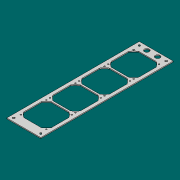
# Autodesk Inventor part: front_panel
Saved by Autodesk Inventor 2018.2 (Build 222227000, 227)
## iProperties
Created: 2019-10-14
Part Number: front_panel
Material: アルミニウム 6061
Document SubType Name: Modeling
Designer: gisen
Density: 2.7 g/cm^3
Appearance: アルミニウム - フラット
Author: gisen
Autodesk Inventor part; units mm, degrees
ref_plane "YZ Plane" through (0, 0, 0) normal (1, 0, 0) x (0, 1, 0)
ref_plane "XZ Plane" through (0, 0, 0) normal (0, 1, 0) x (-1, 0, 0)
ref_plane "XY Plane" through (0, 0, 0) normal (0, 0, 1) x (1, 0, 0)
sketch "スケッチ1" plane through (0, 0, 0) normal (0, 0, 1) x (1, 0, 0)
  line L0 (-55, -215) -> (55, -215)
  line L1 (55, -215) -> (55, 215)
  line L2 (55, 215) -> (-55, 215)
  line L3 (-55, 215) -> (-55, -215)
  line L4 (-55, -215) -> (55, 215) construction
  line L5 (55, -215) -> (-55, 215) construction
  line L6 (-55, 185) -> (-50, 185) construction
  line L7 (-50, 185) -> (-25, 210) construction
  line L8 (-25, 210) -> (-25, 215) construction
  line L9 (-46, 95.75) -> (46, 95.75) construction
  line L10 (46, 95.75) -> (46, 187.75) construction
  line L11 (46, 187.75) -> (-46, 187.75) construction
  line L12 (-46, 187.75) -> (-46, 95.75) construction
  line L13 (-46, 95.75) -> (46, 187.75) construction
  line L14 (46, 95.75) -> (-46, 187.75) construction
  line L15 (-46, 1.25) -> (46, 1.25) construction
  line L16 (46, 1.25) -> (46, 93.25) construction
  line L17 (46, 93.25) -> (-46, 93.25) construction
  line L18 (-46, 93.25) -> (-46, 1.25) construction
  line L19 (-46, 1.25) -> (46, 93.25) construction
  line L20 (46, 1.25) -> (-46, 93.25) construction
  line L21 (0, 0) -> (0, 141.75) construction
  circle A0 centre (0, 141.75) radius 53 construction
  line L22 (-44.7, 97.05) -> (44.7, 97.05) construction
  line L23 (44.7, 97.05) -> (44.7, 186.45) construction
  line L24 (44.7, 186.45) -> (-44.7, 186.45) construction
  line L25 (-44.7, 186.45) -> (-44.7, 97.05) construction
  line L26 (-44.7, 97.05) -> (44.7, 186.45) construction
  line L27 (44.7, 97.05) -> (-44.7, 186.45) construction
  arc A1 (-28.4765, 186.45) -> (-44.7, 170.2265) centre (0, 141.75) ccw
  arc A2 (-44.7, 113.2735) -> (-28.4765, 97.05) centre (0, 141.75) ccw
  arc A3 (28.4765, 97.05) -> (44.7, 113.2735) centre (0, 141.75) ccw
  arc A4 (44.7, 170.2265) -> (28.4765, 186.45) centre (0, 141.75) ccw
  line L28 (-28.4765, 186.45) -> (28.4765, 186.45)
  line L29 (-44.7, 170.2265) -> (-44.7, 113.2735)
  line L30 (-28.4765, 97.05) -> (28.4765, 97.05)
  line L31 (44.7, 113.2735) -> (44.7, 170.2265)
  line L32 (-41.25, 100.5) -> (41.25, 100.5) construction
  line L33 (41.25, 100.5) -> (41.25, 183) construction
  line L34 (41.25, 183) -> (-41.25, 183) construction
  line L35 (-41.25, 183) -> (-41.25, 100.5) construction
  line L36 (-41.25, 100.5) -> (41.25, 183) construction
  line L37 (41.25, 100.5) -> (-41.25, 183) construction
  circle A5 centre (-41.25, 183) radius 2.25
  circle A6 centre (-41.25, 100.5) radius 2.25
  circle A7 centre (41.25, 100.5) radius 2.25
  circle A8 centre (41.25, 183) radius 2.25
  circle A9 centre (-41.25, 88.5) radius 2.25
  arc A10 (-28.4765, 91.95) -> (-44.7, 75.7265) centre (0, 47.25) ccw
  line L38 (-28.4765, 91.95) -> (28.4765, 91.95)
  arc A11 (44.7, 75.7265) -> (28.4765, 91.95) centre (0, 47.25) ccw
  circle A12 centre (41.25, 88.5) radius 2.25
  line L39 (44.7, 18.7735) -> (44.7, 75.7265)
  arc A13 (28.4765, 2.55) -> (44.7, 18.7735) centre (0, 47.25) ccw
  circle A14 centre (41.25, 6) radius 2.25
  line L40 (-28.4765, 2.55) -> (28.4765, 2.55)
  circle A15 centre (-41.25, 6) radius 2.25
  arc A16 (-44.7, 18.7735) -> (-28.4765, 2.55) centre (0, 47.25) ccw
  line L41 (-44.7, 75.7265) -> (-44.7, 18.7735)
  circle A17 centre (-41.25, -6) radius 2.25
  arc A18 (-28.4765, -2.55) -> (-44.7, -18.7735) centre (0, -47.25) ccw
  line L42 (-28.4765, -2.55) -> (28.4765, -2.55)
  arc A19 (44.7, -18.7735) -> (28.4765, -2.55) centre (0, -47.25) ccw
  circle A20 centre (41.25, -6) radius 2.25
  line L43 (44.7, -75.7265) -> (44.7, -18.7735)
  arc A21 (28.4765, -91.95) -> (44.7, -75.7265) centre (0, -47.25) ccw
  circle A22 centre (41.25, -88.5) radius 2.25
  line L44 (-28.4765, -91.95) -> (28.4765, -91.95)
  circle A23 centre (-41.25, -88.5) radius 2.25
  arc A24 (-44.7, -75.7265) -> (-28.4765, -91.95) centre (0, -47.25) ccw
  line L45 (-44.7, -18.7735) -> (-44.7, -75.7265)
  circle A25 centre (-41.25, -100.5) radius 2.25
  arc A26 (-28.4765, -97.05) -> (-44.7, -113.2735) centre (0, -141.75) ccw
  line L46 (-28.4765, -97.05) -> (28.4765, -97.05)
  arc A27 (44.7, -113.2735) -> (28.4765, -97.05) centre (0, -141.75) ccw
  circle A28 centre (41.25, -100.5) radius 2.25
  line L47 (44.7, -170.2265) -> (44.7, -113.2735)
  arc A29 (28.4765, -186.45) -> (44.7, -170.2265) centre (0, -141.75) ccw
  circle A30 centre (41.25, -183) radius 2.25
  line L48 (-28.4765, -186.45) -> (28.4765, -186.45)
  circle A31 centre (-41.25, -183) radius 2.25
  arc A32 (-44.7, -170.2265) -> (-28.4765, -186.45) centre (0, -141.75) ccw
  line L49 (-44.7, -113.2735) -> (-44.7, -170.2265)
  circle A33 centre (-45, 205) radius 2.25
  circle A34 centre (45, 205) radius 2.25
  circle A35 centre (45, -205) radius 2.25
  circle A36 centre (-45, -205) radius 2.25
  circle A37 centre (-45, 0) radius 2.25
  circle A38 centre (45, 0) radius 2.25
  line L50 (-55, 0) -> (55, 0) construction
  point P0 (0, 47.25)
  point P1 (0, 47.25)
  dimension "d12" = 106
  dimension "d0" = 110
  dimension "d1" = 430
  dimension "d2" = 135
  dimension "d3" = 30
  dimension "d4" = 30
  dimension "d5" = 5
  dimension "d6" = 92
  dimension "d7" = 92
  dimension "d8" = 92
  dimension "d9" = 92
  dimension "d10" = 2.5
  dimension "d11" = 1.25
  dimension "d13" = 89.4
  dimension "d14" = 89.4
  dimension "d15" = 82.5
  dimension "d16" = 82.5
  dimension "d17" = 4.5
  dimension "d20" = 94.5
  dimension "d25" = 4.5
  dimension "d26" = 10
  dimension "d27" = 10
  dimension "d28" = 10
  dimension "d29" = 10
  dimension "d30" = 10
  dimension "d31" = 10
  dimension "d32" = 10
  dimension "d33" = 10
  dimension "d34" = 10
  dimension "d35" = 10
  constraints: 102 end point, 38 centre point, 32 point on circle, 18 coincident, 13 midpoint, 13 point on line, 10 parallel, 8 equal radius, 8 perpendicular, 6 horizontal, 2 vertical, 1 collinear, 94 other
  measures "d0" distance of L2.end L1.end
  measures "d1" distance of L1.end L0.end
  measures "d2" angle of L7 L6
  measures "d3" distance between parallel lines of L8 L3
  measures "d4" distance between parallel lines of L2 L6
  measures "d5" distance of L7.end L8.end
  measures "d6" distance of L11.end L10.end
  measures "d7" distance of L10.end L9.end
  measures "d8" distance of L17.end L16.end
  measures "d9" distance of L16.end L15.end
  measures "d10" distance between parallel lines of L17 L9
  measures "d11" distance from line of L21.start L15
  measures "d13" distance of L24.end L23.end
  measures "d14" distance of L23.end L22.end
  measures "d15" distance of L34.end L33.end
  measures "d16" distance of L33.end L32.end
  measures "d17" diameter of A5
  measures "d20" distance of A5.centre A9.centre
  measures "d25" diameter of A33
  measures "d26" distance from line of A33.centre L2
  measures "d27" distance from line of L3 A33.centre
  measures "d28" distance from line of L2 A34.centre
  measures "d29" distance from line of L1 A34.centre
  measures "d30" distance from line of L1 A35.centre
  measures "d31" distance from line of L0 A35.centre
  measures "d32" distance from line of L0 A36.centre
  measures "d33" distance from line of L3 A36.centre
  measures "d34" distance from line of L3 A37.centre
  measures "d35" distance from line of L1 A38.centre
extrude "押し出し1" add sketch "スケッチ1" along normal blind 3 contours L3 L2 L1 L0 | A37 | A38
sketch "スケッチ2" plane through (0, 0, 3) normal (0, 0, 1) x (1, 0, 0)
  circle A0 centre (-45, 205) radius 2.25 construction
  circle A1 centre (45, -205) radius 2.25 construction
  circle A2 centre (-45, -205) radius 2.25 construction
  circle A3 centre (-43, 203) radius 2.75 construction
  line L0 (55, 215) -> (-55, 215) projected
  line L1 (-55, 215) -> (-55, -215) projected
  line L2 (-43.7153, 206.8472) -> (-41.4298, 205.2577)
  line L3 (-45.2577, 201.4298) -> (-46.8472, 203.7153)
  circle A4 centre (-45, 205) radius 2.25 construction
  arc A5 (-43.7153, 206.8472) -> (-46.8472, 203.7153) centre (-45, 205) ccw
  arc A6 (-45.2577, 201.4298) -> (-41.4298, 205.2577) centre (-43, 203) ccw
  line L4 (55, 215) -> (-55, 215) construction
  line L5 (0, 215) -> (0, -215) construction
  line L6 (-55, -215) -> (55, -215) construction
  line L7 (-55, 0) -> (55, 0) construction
  line L8 (55, -215) -> (55, 215) construction
  circle A7 centre (45, 205) radius 2.25 construction
  circle A8 centre (43, 203) radius 2.75 construction
  line L9 (43.7153, 206.8472) -> (41.4298, 205.2577)
  line L10 (45.2577, 201.4298) -> (46.8472, 203.7153)
  circle A9 centre (45, 205) radius 2.25 construction
  arc A10 (46.8472, 203.7153) -> (43.7153, 206.8472) centre (45, 205) ccw
  arc A11 (41.4298, 205.2577) -> (45.2577, 201.4298) centre (43, 203) ccw
  circle A12 centre (-45, -205) radius 2.25 construction
  circle A13 centre (-43, -203) radius 2.75 construction
  line L11 (-43.7153, -206.8472) -> (-41.4298, -205.2577)
  line L12 (-45.2577, -201.4298) -> (-46.8472, -203.7153)
  circle A14 centre (-45, -205) radius 2.25 construction
  arc A15 (-46.8472, -203.7153) -> (-43.7153, -206.8472) centre (-45, -205) ccw
  arc A16 (-41.4298, -205.2577) -> (-45.2577, -201.4298) centre (-43, -203) ccw
  circle A17 centre (45, -205) radius 2.25 construction
  line L13 (45.2577, -201.4298) -> (46.8472, -203.7153)
  arc A18 (45.2577, -201.4298) -> (41.4298, -205.2577) centre (43, -203) ccw
  circle A19 centre (43, -203) radius 2.75 construction
  line L14 (43.7153, -206.8472) -> (41.4298, -205.2577)
  circle A20 centre (45, -205) radius 2.25 construction
  arc A21 (43.7153, -206.8472) -> (46.8472, -203.7153) centre (45, -205) ccw
  point P0 (0, 0)
  dimension "d38" = 5.5
  dimension "d39" = 12
  dimension "d40" = 12
  constraints: 28 point on circle, 27 symmetric about line, 20 end point, 15 centre point, 8 coincident, 4 midpoint, 2 horizontal, 2 tangent, 1 vertical, 25 other
  measures "d38" diameter of A3
  measures "d39" distance from line of A3.centre L0
  measures "d40" distance from line of L1 A3.centre
extrude "押し出し2" cut sketch "スケッチ2" against normal through all
sketch "スケッチ4" plane through (0, 0, 3) normal (0, 0, 1) x (1, 0, 0)
  line L0 (55, 215) -> (-55, 215) construction
  line L1 (-28.4765, 186.45) -> (28.4765, 186.45) construction
  line L2 (55, 215) -> (-55, 215) construction
  line L3 (0, 215) -> (0, 186.45) construction
  arc A0 (-19.9739, 209.45) -> (-19.9739, 194.55) centre (-17.5, 202) ccw construction
  line L4 (-19.9739, 209.45) -> (-15.0261, 209.45) construction
  line L5 (-15.0261, 194.55) -> (-19.9739, 194.55) construction
  arc A1 (-15.0261, 209.45) -> (-19.9739, 209.45) centre (-17.5, 202) ccw construction
  arc A2 (-15.0261, 194.55) -> (-15.0261, 209.45) centre (-17.5, 202) ccw construction
  arc A3 (-19.9739, 194.55) -> (-15.0261, 194.55) centre (-17.5, 202) ccw construction
  line L6 (-19.9755, 194.54) -> (-15.0245, 194.54)
  arc A4 (-15.0245, 194.54) -> (-15.0245, 209.46) centre (-17.5, 202) ccw
  line L7 (-15.0245, 209.46) -> (-19.9755, 209.46)
  arc A5 (-19.9755, 209.46) -> (-19.9755, 194.54) centre (-17.5, 202) ccw
  line L8 (-25, 215) -> (-25, 210) construction
  line L9 (-25, 210) -> (-50, 185) construction
  line L10 (-50, 185) -> (-55, 185) construction
  line L11 (-55, 215) -> (-55, -215) construction
  line L12 (19.9755, 194.54) -> (15.0245, 194.54)
  line L13 (15.0245, 209.46) -> (19.9755, 209.46)
  arc A6 (15.0245, 209.46) -> (15.0245, 194.54) centre (17.5, 202) ccw
  arc A7 (19.9755, 194.54) -> (19.9755, 209.46) centre (17.5, 202) ccw
  point P0 (0, 0)
  dimension "d46" = 15.7
  dimension "d47" = 14.9
  dimension "d48" = 0.01
  dimension "d49" = 13
  dimension "d50" = 17.5
  dimension "d51" = 135
  dimension "d52" = 30
  dimension "d53" = 5
  constraints: 20 end point, 17 point on circle, 8 centre point, 5 symmetric about line, 2 equal length, 2 midpoint, 2 parallel, 2 perpendicular, 2 point on line, 1 horizontal, 5 other
  measures "d46" diameter of A0
  measures "d47" distance between parallel lines of L5 L4
  measures "d48" radial gap between concentric circles of A0 A5
  measures "d49" distance from line of A3.centre L0
  measures "d50" distance from line of L3 A3.centre
  measures "d51" angle of L8 L9
  measures "d52" distance between parallel lines of L8 L11
  measures "d53" distance of L9.end L10.end
extrude "押し出し4" cut sketch "スケッチ4" against normal through all
sketch "スケッチ3" plane through (0, 0, 0) normal (0, 0, -1) x (-1, 0, 0)
  line L0 (-55, 215) -> (55, 215) construction
  line L1 (-55, -215) -> (-55, 215) construction
  line L2 (55, -215) -> (-55, -215) construction
  line L3 (55, 215) -> (55, -215) construction
  line L4 (54.75, 214.75) -> (-54.75, 214.75)
  line L5 (-54.75, 214.75) -> (-54.75, -214.75)
  line L6 (-54.75, -214.75) -> (54.75, -214.75)
  line L7 (54.75, -214.75) -> (54.75, 214.75)
  point P0 (0, 0)
  dimension "d43" = 0.25
  constraints: 8 end point, 3 other
  measures "d43" distance between parallel lines of L0 L4
extrude "押し出し3" [suppressed]
equation "\"d4\" = d3"
equation "\"d11\" = 0.5 * d10"
equation "\"d20\" = d7 + d10"
equation "\"d27\" = d26"
equation "\"d28\" = d26"
equation "\"d29\" = d26"
equation "\"d30\" = d26"
equation "\"d31\" = d26"
equation "\"d32\" = d26"
equation "\"d33\" = d26"
equation "\"d34\" = d26"
equation "\"d35\" = d26"
